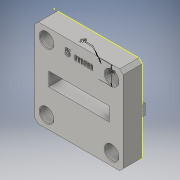
# Autodesk Inventor part: Cage Plate Slit 5mm
Saved by Autodesk Inventor 2016 (Build 200138000, 138)
## iProperties
Created: 2015-08-27
Part Number: Cage Plate Slit 5mm
Material: Generic
Document SubType Name: Modeling
Designer: kthorn
Density: 1 g/cm^3
Appearance: Default
Author: kthorn
Autodesk Inventor part; units mm, degrees
ref_plane "YZ Plane" through (0, 0, 0) normal (1, 0, 0) x (0, 1, 0)
ref_plane "XZ Plane" through (0, 0, 0) normal (0, 1, 0) x (-1, 0, 0)
ref_plane "XY Plane" through (0, 0, 0) normal (0, 0, 1) x (1, 0, 0)
sketch "Sketch1" plane through (0, 0, 0) normal (0, 0, 1) x (1, 0, 0)
  line L0 (1.5875, 0) -> (39.0525, 0)
  line L1 (40.64, -1.5875) -> (40.64, -39.0525)
  line L2 (39.0525, -40.64) -> (1.5875, -40.64)
  line L3 (0, -39.0525) -> (0, -1.5875)
  line L4 (5.3213, -5.3213) -> (35.3187, -5.3213) construction
  line L5 (35.3187, -5.3213) -> (35.3187, -35.3187) construction
  line L6 (35.3187, -35.3187) -> (5.3213, -35.3187) construction
  line L7 (5.3213, -35.3187) -> (5.3213, -5.3213) construction
  line L8 (35.3187, -5.3213) -> (40.64, 0) construction
  line L9 (5.3213, -35.3187) -> (0, -40.64) construction
  line L10 (5.3213, -5.3213) -> (0, 0) construction
  circle A0 centre (5.3213, -5.3213) radius 3.175
  circle A1 centre (35.3187, -5.3213) radius 3.175
  circle A2 centre (35.3187, -35.3187) radius 3.175
  circle A3 centre (5.3213, -35.3187) radius 3.175
  line L11 (1.5875, 0) -> (0, -1.5875)
  line L12 (0, -39.0525) -> (1.5875, -40.64)
  line L13 (39.0525, 0) -> (40.64, -1.5875)
  line L14 (40.64, -39.0525) -> (39.0525, -40.64)
  point P0 (40.64, -40.64)
  point P1 (40.64, -40.64)
  dimension "d0" = 40.64
  dimension "d1" = 29.9974
  dimension "d2" = 6.35
  dimension "d3" = 1.5875
  dimension "d4" = 1.5875
  dimension "d5" = 1.5875
  dimension "d6" = 1.5875
  dimension "d7" = 1.5875
  dimension "d8" = 1.5875
  dimension "d11" = 1.5875
  dimension "d12" = 1.5875
  constraints: 30 end point, 10 point on line, 6 perpendicular, 5 coincident, 4 centre point, 4 parallel, 3 equal radius, 2 horizontal
  measures "d0" distance of L10.end L8.end
  measures "d1" distance of L4.start L4.end
  measures "d2" diameter of A0
  measures "d3" distance of L0.start L10.end
  measures "d4" distance of L3.end L10.end
  measures "d5" distance of L3.start L9.end
  measures "d6" distance of L2.end L9.end
  measures "d7" distance of L0.end L8.end
  measures "d8" distance of L1.start L8.end
  measures "d11" distance of L1.end point (40.64, -40.64)
  measures "d12" distance of L2.start point (40.64, -40.64)
extrude "Extrusion1" add sketch "Sketch1" along normal blind 8.89
sketch "Sketch2" plane through (0, 0, 8.89) normal (0, 0, 1) x (1, 0, 0)
  circle A0 centre (5.3213, -35.3187) radius 3.175 projected
  circle A1 centre (35.3187, -35.3187) radius 3.175 projected
  circle A2 centre (35.3187, -5.3213) radius 3.175 projected
  circle A3 centre (5.3213, -5.3213) radius 3.175 projected
  line L0 (1.5875, 0) -> (0, -1.5875) projected
  line L1 (0, -1.5875) -> (0, -39.0525) projected
  line L2 (0, -39.0525) -> (1.5875, -40.64) projected
  line L3 (1.5875, -40.64) -> (39.0525, -40.64) projected
  line L4 (39.0525, -40.64) -> (40.64, -39.0525) projected
  line L5 (40.64, -39.0525) -> (40.64, -1.5875) projected
  line L6 (40.64, -1.5875) -> (39.0525, 0) projected
  line L7 (39.0525, 0) -> (1.5875, 0) projected
  line L8 (6.35, -20.32) -> (0, -20.32) construction
  line L9 (0, -1.5875) -> (0, -39.0525) projected
  line L10 (34.29, -20.32) -> (40.64, -20.32) construction
  line L11 (40.64, -39.0525) -> (40.64, -1.5875) projected
  line L12 (6.35, -17.145) -> (34.29, -17.145)
  line L13 (34.29, -17.145) -> (34.29, -23.495)
  line L14 (34.29, -23.495) -> (6.35, -23.495)
  line L15 (6.35, -23.495) -> (6.35, -17.145)
  line L16 (34.29, -23.495) -> (40.64, -23.495) construction
  point P0 (0, 0)
  dimension "d17" = 6.35
  dimension "d18" = 27.94
  constraints: 14 end point, 4 midpoint, 2 horizontal, 2 parallel, 2 perpendicular, 1 collinear, 1 point on line
  measures "d17" distance of L12.end L13.end
  measures "d18" distance of L13.end L14.end
sketch "Sketch3" plane through (0, 0, 8.89) normal (0, 0, 1) x (1, 0, 0)
  line L0 (9.5396, -2.9704) -> (31.1004, -2.9704) construction
  line L1 (31.1004, -2.9704) -> (31.1004, -7.6722) construction
  line L2 (31.1004, -7.6722) -> (9.5396, -7.6722) construction
  line L3 (9.5396, -7.6722) -> (9.5396, -2.9704) construction
  line L4 (37.465, 0) -> (0, 0)
  line L5 (0, 0) -> (0, -8.89)
  line L6 (37.465, -8.89) -> (0, -8.89)
  line L7 (37.465, 0) -> (37.465, -8.89)
  circle A0 centre (35.3187, -5.3213) radius 3.175 construction
  line L8 (35.3187, -5.3213) -> (31.1004, -5.3213) construction
  circle A1 centre (5.3213, -5.3213) radius 3.175 construction
  line L9 (5.3213, -5.3213) -> (9.5396, -5.3213) construction
  line L10 (14.2038, -3.7063) -> (16.294, -3.7063)
  line L11 (16.294, -3.7063) -> (16.294, -4.4091)
  line L12 (16.294, -4.4091) -> (14.8791, -4.4091)
  line L13 (14.8791, -4.4091) -> (14.8058, -4.8858)
  spline S0 degree 2 poles (14.8058, -4.8858) (14.9524, -4.8186) (15.2397, -4.7483) (15.3803, -4.7483) knots 0 0 0 1 2 2 2
  spline S1 degree 2 poles (15.3803, -4.7483) (15.8539, -4.7483) (16.4467, -5.3259) (16.4467, -5.7629) knots 0 0 0 1 2 2 2
  spline S2 degree 2 poles (16.4467, -5.7629) (16.4467, -6.0684) (16.1412, -6.6368) (15.5819, -6.9363) (15.145, -6.9363) knots 0 0 0 1 2 3 3 3
  spline S3 degree 2 poles (15.145, -6.9363) (14.8302, -6.9363) (14.3841, -6.8171) (14.0693, -6.5818) (13.8737, -6.2824) (13.8096, -6.0593) knots 0 0 0 1 2 3 4 4 4
  line L14 (13.8096, -6.0593) -> (14.7019, -5.9615)
  spline S4 degree 2 poles (14.7019, -5.9615) (14.7355, -6.1754) (14.9708, -6.3985) (15.1358, -6.3985) knots 0 0 0 1 2 2 2
  spline S5 degree 2 poles (15.1358, -6.3985) (15.3191, -6.3985) (15.5575, -6.1204) (15.5575, -5.8423) knots 0 0 0 1 2 2 2
  spline S6 degree 2 poles (15.5575, -5.8423) (15.5575, -5.5581) (15.3161, -5.2953) (15.1175, -5.2953) knots 0 0 0 1 2 2 2
  spline S7 degree 2 poles (15.1175, -5.2953) (14.9891, -5.2953) (14.8699, -5.3595) knots 0 0 0 1 1 1
  spline S8 degree 2 poles (14.8699, -5.3595) (14.7844, -5.4023) (14.6774, -5.5215) knots 0 0 0 1 1 1
  line L15 (14.6774, -5.5215) -> (13.9257, -5.4145)
  line L16 (13.9257, -5.4145) -> (14.2038, -3.7063)
  line L17 (18.375, -4.5803) -> (19.197, -4.5803)
  line L18 (19.197, -4.5803) -> (19.197, -4.9164)
  spline S9 degree 2 poles (19.197, -4.9164) (19.3742, -4.7056) (19.7379, -4.5283) (19.9946, -4.5283) knots 0 0 0 1 2 2 2
  spline S10 degree 2 poles (19.9946, -4.5283) (20.2696, -4.5283) (20.5904, -4.7239) (20.6913, -4.9164) knots 0 0 0 1 2 2 2
  spline S11 degree 2 poles (20.6913, -4.9164) (20.8991, -4.6903) (21.2413, -4.5283) (21.4919, -4.5283) knots 0 0 0 1 2 2 2
  spline S12 degree 2 poles (21.4919, -4.5283) (21.8617, -4.5283) (22.2773, -4.9684) (22.2773, -5.4359) knots 0 0 0 1 2 2 2
  line L19 (22.2773, -5.4359) -> (22.2773, -6.8813)
  line L20 (22.2773, -6.8813) -> (21.3941, -6.8813)
  line L21 (21.3941, -6.8813) -> (21.3941, -5.5703)
  spline S13 degree 2 poles (21.3941, -5.5703) (21.3941, -5.4145) (21.333, -5.3381) knots 0 0 0 1 1 1
  spline S14 degree 2 poles (21.333, -5.3381) (21.2444, -5.2189) (21.113, -5.2189) knots 0 0 0 1 1 1
  spline S15 degree 2 poles (21.113, -5.2189) (20.9571, -5.2189) (20.7677, -5.4451) (20.7677, -5.6926) knots 0 0 0 1 2 2 2
  line L22 (20.7677, -5.6926) -> (20.7677, -6.8813)
  line L23 (20.7677, -6.8813) -> (19.8845, -6.8813)
  line L24 (19.8845, -6.8813) -> (19.8845, -5.6131)
  spline S16 degree 2 poles (19.8845, -5.6131) (19.8845, -5.4634) (19.8662, -5.4084) knots 0 0 0 1 1 1
  spline S17 degree 2 poles (19.8662, -5.4084) (19.8387, -5.3228) (19.7012, -5.2159) (19.6065, -5.2159) knots 0 0 0 1 2 2 2
  spline S18 degree 2 poles (19.6065, -5.2159) (19.4537, -5.2159) (19.2581, -5.4451) (19.2581, -5.7079) knots 0 0 0 1 2 2 2
  line L25 (19.2581, -5.7079) -> (19.2581, -6.8813)
  line L26 (19.2581, -6.8813) -> (18.375, -6.8813)
  line L27 (18.375, -6.8813) -> (18.375, -4.5803)
  line L28 (22.812, -4.5803) -> (23.634, -4.5803)
  line L29 (23.634, -4.5803) -> (23.634, -4.9164)
  spline S19 degree 2 poles (23.634, -4.9164) (23.8113, -4.7056) (24.1749, -4.5283) (24.4316, -4.5283) knots 0 0 0 1 2 2 2
  spline S20 degree 2 poles (24.4316, -4.5283) (24.7066, -4.5283) (25.0275, -4.7239) (25.1283, -4.9164) knots 0 0 0 1 2 2 2
  spline S21 degree 2 poles (25.1283, -4.9164) (25.3361, -4.6903) (25.6784, -4.5283) (25.929, -4.5283) knots 0 0 0 1 2 2 2
  spline S22 degree 2 poles (25.929, -4.5283) (26.2987, -4.5283) (26.7143, -4.9684) (26.7143, -5.4359) knots 0 0 0 1 2 2 2
  line L30 (26.7143, -5.4359) -> (26.7143, -6.8813)
  line L31 (26.7143, -6.8813) -> (25.8312, -6.8813)
  line L32 (25.8312, -6.8813) -> (25.8312, -5.5703)
  spline S23 degree 2 poles (25.8312, -5.5703) (25.8312, -5.4145) (25.7701, -5.3381) knots 0 0 0 1 1 1
  spline S24 degree 2 poles (25.7701, -5.3381) (25.6814, -5.2189) (25.55, -5.2189) knots 0 0 0 1 1 1
  spline S25 degree 2 poles (25.55, -5.2189) (25.3942, -5.2189) (25.2047, -5.4451) (25.2047, -5.6926) knots 0 0 0 1 2 2 2
  line L33 (25.2047, -5.6926) -> (25.2047, -6.8813)
  line L34 (25.2047, -6.8813) -> (24.3216, -6.8813)
  line L35 (24.3216, -6.8813) -> (24.3216, -5.6131)
  spline S26 degree 2 poles (24.3216, -5.6131) (24.3216, -5.4634) (24.3033, -5.4084) knots 0 0 0 1 1 1
  spline S27 degree 2 poles (24.3033, -5.4084) (24.2758, -5.3228) (24.1383, -5.2159) (24.0435, -5.2159) knots 0 0 0 1 2 2 2
  spline S28 degree 2 poles (24.0435, -5.2159) (23.8907, -5.2159) (23.6952, -5.4451) (23.6952, -5.7079) knots 0 0 0 1 2 2 2
  line L36 (23.6952, -5.7079) -> (23.6952, -6.8813)
  line L37 (23.6952, -6.8813) -> (22.812, -6.8813)
  line L38 (22.812, -6.8813) -> (22.812, -4.5803)
  point P0 (-1.5875, 0)
  constraints: 12 end point, 2 horizontal, 2 midpoint, 1 collinear, 2 other
extrude "Extrusion4" cut sketch "Sketch3" against normal blind 0.889 contours L10 L11 L12 L13 S0 S1 S2 S3 L14 S4 S5 S6 S7 S8 L15 L16 | L17 L18 S9 S10 S11 S12 L19 L20 L21 S13 S14 S15 L22 L23 L24 S16 S17 S18 L25 L26 L27 | L28 L29 S19 S20 S21 S22 L30 L31 L32 S23 S24 S25 L33 L34 L35 S26 S27 S28 L36 L37 L38
extrude "Extrusion8" cut sketch "Sketch2" against normal through all contours L12 L13 L14 L15
sketch "Sketch4" plane through (0, 0, 0) normal (0, 0, -1) x (-1, 0, 0)
  circle A0 centre (-5.3213, -35.3187) radius 3.175 projected
  circle A1 centre (-35.3187, -35.3187) radius 3.175 projected
  circle A2 centre (-35.3187, -5.3213) radius 3.175 projected
  circle A3 centre (-5.3213, -5.3213) radius 3.175 projected
  line L0 (-1.5875, 0) -> (0, -1.5875) projected
  line L1 (-39.0525, 0) -> (-1.5875, 0) projected
  line L2 (-40.64, -1.5875) -> (-39.0525, 0) projected
  line L3 (-40.64, -39.0525) -> (-40.64, -1.5875) projected
  line L4 (-39.0525, -40.64) -> (-40.64, -39.0525) projected
  line L5 (-1.5875, -40.64) -> (-39.0525, -40.64) projected
  line L6 (0, -39.0525) -> (-1.5875, -40.64) projected
  line L7 (0, -1.5875) -> (0, -39.0525) projected
  line L8 (0, -1.5875) -> (0, -39.0525) projected
  line L9 (-40.64, -22.82) -> (-34.29, -22.82)
  line L10 (-34.29, -22.82) -> (-34.29, -17.82)
  line L11 (-34.29, -17.82) -> (-40.64, -17.82)
  line L12 (-40.64, -17.82) -> (-40.64, -22.82)
  line L13 (-39.0525, 0) -> (-1.5875, 0) construction
  line L14 (-20.32, 0) -> (-20.32, -40.64) construction
  line L15 (-1.5875, -40.64) -> (-39.0525, -40.64) construction
  line L16 (0, -22.82) -> (-6.35, -22.82)
  line L17 (-6.35, -22.82) -> (-6.35, -17.82)
  line L18 (-6.35, -17.82) -> (0, -17.82)
  line L19 (0, -17.82) -> (0, -22.82)
  line L20 (-34.29, -23.495) -> (-34.29, -17.145) projected
  line L21 (-6.35, -17.145) -> (-6.35, -23.495) projected
  point P0 (0, 0)
  point P1 (-40.64, -20.32)
  point P2 (0, -20.32)
  point P3 (-34.29, -20.32)
  dimension "d45" = 5
  dimension "d48" = 27.94
  constraints: 18 end point, 6 midpoint, 5 symmetric about line, 2 parallel, 1 horizontal, 1 perpendicular
  measures "d45" distance of L9.end L10.end
  measures "d48" distance of L18.start L10.end
extrude "Extrusion5" add sketch "Sketch4" along normal blind 1.27 contours L7 L16 L17 L18 | L11 L10 L9 L3
sketch "Sketch5" plane through (0, 0, 0) normal (0, 0, -1) x (-1, 0, 0)
  line L0 (0, -1.5875) -> (0, -17.82) projected
  line L1 (-1.5875, 0) -> (0, -1.5875) projected
  line L2 (-39.0525, 0) -> (-1.5875, 0) projected
  line L3 (-40.64, -1.5875) -> (-39.0525, 0) projected
  line L4 (-40.64, -39.0525) -> (-40.64, -22.82) projected
  circle A0 centre (-35.3187, -5.3213) radius 3.175 projected
  circle A1 centre (-5.3213, -5.3213) radius 3.175 projected
  circle A2 centre (-35.3187, -35.3187) radius 3.175 projected
  circle A3 centre (-5.3213, -35.3187) radius 3.175 projected
  line L5 (-40.64, -39.0525) -> (-40.64, -22.82) projected
  line L6 (-39.0525, -40.64) -> (-40.64, -39.0525) projected
  line L7 (-1.5875, -40.64) -> (-39.0525, -40.64) projected
  line L8 (0, -39.0525) -> (-1.5875, -40.64) projected
  line L9 (0, -1.5875) -> (0, -17.82) projected
  line L10 (-20.32, -17.82) -> (-20.32, -9.184) construction
  circle A4 centre (-20.32, -9.184) radius 1.7145
  circle A5 centre (-20.32, -9.184) radius 2.413
  line L11 (0, -1.5875) -> (0, -39.0525) construction
  line L12 (-40.64, -39.0525) -> (-40.64, -1.5875) construction
  line L13 (-1.5875, 0) -> (0, -1.5875) projected
  line L14 (-39.0525, 0) -> (-1.5875, 0) projected
  line L15 (-40.64, -1.5875) -> (-39.0525, 0) projected
  line L16 (-39.0525, -40.64) -> (-40.64, -39.0525) projected
  line L17 (-1.5875, -40.64) -> (-39.0525, -40.64) projected
  line L18 (0, -39.0525) -> (-1.5875, -40.64) projected
  line L19 (-34.29, -22.82) -> (-40.64, -22.82) projected
  line L20 (0, -22.82) -> (0, -39.0525) projected
  line L21 (0, -22.82) -> (-6.35, -22.82) projected
  line L22 (-6.35, -22.82) -> (-6.35, -23.495) projected
  line L23 (-6.35, -23.495) -> (-34.29, -23.495) projected
  line L24 (-34.29, -23.495) -> (-34.29, -22.82) projected
  line L25 (-40.64, -17.82) -> (-34.29, -17.82) projected
  line L26 (-34.29, -17.82) -> (-34.29, -17.145) projected
  line L27 (-34.29, -17.145) -> (-6.35, -17.145) projected
  line L28 (-6.35, -17.145) -> (-6.35, -17.82) projected
  line L29 (-6.35, -17.82) -> (0, -17.82) projected
  line L30 (-40.64, -17.82) -> (-40.64, -1.5875) projected
  line L31 (-34.29, -22.82) -> (-40.64, -22.82) projected
  line L32 (0, -22.82) -> (0, -39.0525) projected
  line L33 (0, -22.82) -> (-6.35, -22.82) projected
  line L34 (-6.35, -22.82) -> (-6.35, -23.495) projected
  line L35 (-6.35, -23.495) -> (-34.29, -23.495) projected
  line L36 (-34.29, -23.495) -> (-34.29, -22.82) projected
  line L37 (-40.64, -17.82) -> (-34.29, -17.82) projected
  line L38 (-34.29, -17.82) -> (-34.29, -17.145) projected
  line L39 (-34.29, -17.145) -> (-6.35, -17.145) projected
  line L40 (-6.35, -17.145) -> (-6.35, -17.82) projected
  line L41 (-6.35, -17.82) -> (0, -17.82) projected
  line L42 (-40.64, -17.82) -> (-40.64, -1.5875) projected
  line L43 (-40.64, -17.82) -> (0, -17.82) construction
  line L44 (-40.64, -20.32) -> (0, -20.32) construction
  circle A6 centre (-20.32, -31.456) radius 1.7145
  circle A7 centre (-20.32, -31.456) radius 2.413
  point P0 (0, 0)
  point P1 (-20.32, -29.464)
  dimension "d36" = 8.636
  dimension "d37" = 3.429
  dimension "d38" = 4.826
  constraints: 6 end point, 4 centre point, 4 coincident, 3 midpoint, 3 symmetric about line, 1 perpendicular, 1 vertical, 2 other
  measures "d36" distance of L10.start L10.end
  measures "d37" diameter of A4
  measures "d38" diameter of A5
extrude "Extrusion6" cut sketch "Sketch5" against normal blind 4.318 contours A4 | A6
extrude "Extrusion7" cut sketch "Sketch5" against normal blind 0.508 contours A5 | A6 | A7
chamfer "Chamfer2" distance 0.254 angle 45 4 edges at (32.1437, -5.3213, 0) (32.1437, -35.3187, 0) (2.1463, -35.3187, 0) (2.1463, -5.3213, 0)
chamfer "Chamfer3" distance 0.254 angle 45 4 edges at (32.1437, -5.3213, 8.89) (2.1463, -5.3213, 8.89) (2.1463, -35.3187, 8.89) (32.1437, -35.3187, 8.89)
equation "\"d4\" = d3"
equation "\"d5\" = d3"
equation "\"d6\" = d5"
equation "\"d8\" = d7"
equation "\"d11\" = d9"
equation "\"d12\" = d11"
equation "\"d9\" = 1.5875"
body "Solid1"
